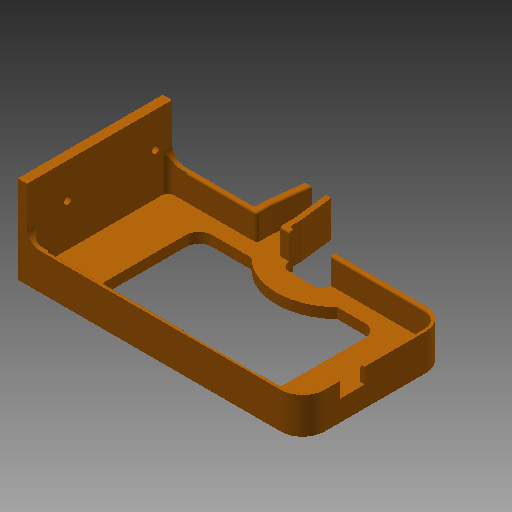
# Autodesk Inventor part: Phone_Cas
Saved by Autodesk Inventor 2019 (Build 230136000, 136)
## iProperties
Created: 2015-11-17
Part Number: Phone_Cas
Material: Generic
Document SubType Name: Modeling
Designer: Team Titanium
Density: 1 g/cm^3
Appearance: Orange
Author: Team Titanium
Autodesk Inventor part; units mm, degrees
ref_plane "YZ Plane" through (0, 0, 0) normal (1, 0, 0) x (0, 1, 0)
ref_plane "XZ Plane" through (0, 0, 0) normal (0, 1, 0) x (-1, 0, 0)
ref_plane "XY Plane" through (0, 0, 0) normal (0, 0, 1) x (1, 0, 0)
sketch "Sketch1" plane through (0, 0, 0) normal (0, 1, 0) x (-1, 0, 0)
  line L0 (67.1674, 24.5628) -> (-66.5636, 24.5628)
  line L1 (-66.5636, 24.5628) -> (-66.5636, -42.8742)
  line L2 (-66.5636, -42.8742) -> (67.1674, -42.8742)
  line L3 (67.1674, -42.8742) -> (67.1674, 24.5628)
  line L4 (69.1994, 26.5948) -> (-68.5956, 26.5948)
  line L5 (-68.5956, 26.5948) -> (-68.5956, -44.9062)
  line L6 (-68.5956, -44.9062) -> (69.1994, -44.9062)
  line L7 (69.1994, -44.9062) -> (69.1994, 26.5948)
  point P0 (0, 0)
  dimension "d0" = 133.731
  dimension "d1" = 67.437
  dimension "d2" = 2.032
  constraints: 16 end point, 4 parallel, 2 perpendicular, 1 horizontal, 3 other
  measures "d0" distance of L1.end L2.end
  measures "d1" distance of L2.end L0.start
  measures "d2" distance between parallel lines of L4 L0
extrude "Extrusion1" add sketch "Sketch1" along normal blind 12.7
sketch "Sketch2" plane through (0, 0, 0) normal (0, -1, 0) x (1, 0, 0)
  line L0 (68.5956, 26.5948) -> (68.5956, -44.9062) projected
  line L1 (68.5956, -44.9062) -> (-69.1994, -44.9062) projected
  line L2 (-69.1994, -44.9062) -> (-69.1994, 26.5948) projected
  line L3 (-69.1994, 26.5948) -> (68.5956, 26.5948) projected
  point P0 (0, 0)
extrude "Extrusion2" add sketch "Sketch2" along normal blind 5.08
fillet "Fillet1" radius 7.62 4 edges at (-67.1674, 6.35, -42.8742) (66.5636, 6.35, -42.8742) (-67.1674, 6.35, 24.5628) (66.5636, 6.35, 24.5628)
fillet "Fillet2" radius 10.795 4 edges at (-69.1994, 3.81, -44.9062) (68.5956, 3.81, -44.9062) (68.5956, 3.81, 26.5948) (-69.1994, 3.81, 26.5948)
sketch "Sketch3" plane through (0, 12.7, 0) normal (0, 1, 0) x (1, 0, 0)
  line L0 (57.8006, 44.9062) -> (-58.4044, 44.9062) projected
  line L1 (-59.5474, 42.8742) -> (58.9436, 42.8742) projected
  line L2 (-23.4286, 44.9062) -> (-12.7606, 44.9062)
  line L3 (-12.7606, 44.9062) -> (-12.7606, 42.8742)
  line L4 (-12.7606, 42.8742) -> (-23.4286, 42.8742)
  line L5 (-23.4286, 42.8742) -> (-23.4286, 44.9062)
  line L6 (-67.1674, -16.9428) -> (-67.1674, 35.2542) projected
  point P0 (0, 0)
  point P1 (-18.0946, 42.8742)
  dimension "d9" = 10.668
  dimension "d50" = 49.0728
  constraints: 8 end point, 2 parallel, 2 point on line, 1 horizontal, 1 midpoint, 1 perpendicular
  measures "d9" distance of L2.start L2.end
  measures "d50" distance from line of point (-18.095, 42.874) L6
extrude "Extrusion3" cut sketch "Sketch3" against normal up to surface (12.7 mm away)
sketch "Sketch4" plane through (0, 12.7, 0) normal (0, 1, 0) x (1, 0, 0)
  line L0 (-12.7606, 44.9062) -> (-12.7606, 50.6847)
  line L1 (-12.7606, 50.6847) -> (-14.8579, 67.7662)
  line L2 (-23.4286, 44.9062) -> (-23.4286, 50.6847)
  line L3 (-23.4286, 50.6847) -> (-21.3312, 67.7662)
  line L4 (-23.4286, 44.9062) -> (-58.4044, 44.9062) projected
  line L5 (-14.8579, 67.7662) -> (-11.6591, 67.7662)
  line L6 (-11.6591, 67.7662) -> (-9.5856, 50.8788)
  line L7 (57.8006, 44.9062) -> (-12.7606, 44.9062) projected
  line L8 (-9.5856, 44.9062) -> (-9.5856, 50.8788)
  line L9 (-21.3312, 67.7662) -> (-24.5301, 67.7662)
  line L10 (-24.5301, 67.7662) -> (-26.6036, 50.8788)
  line L11 (-26.6036, 50.8788) -> (-26.6036, 44.9062)
  line L12 (-67.1674, -16.9428) -> (-67.1674, 35.2542) projected
  point P0 (0, 0)
  dimension "d14" = 5.7785
  dimension "d15" = 22.86
  dimension "d17" = 3.175
  dimension "d18" = 3.175
  dimension "d19" = 3.175
  dimension "d20" = 3.175
  dimension "d45" = 173
  dimension "d46" = 173
  dimension "d47" = 6.4733
  constraints: 20 end point, 2 horizontal, 2 horizontal alignment, 2 perpendicular, 2 point on line, 2 vertical, 1 equal length, 1 parallel
  measures "d14" distance of L2.start L2.end
  measures "d15" distance from line of L3.end L4
  measures "d17" distance between parallel lines of L6 L1
  measures "d18" distance between parallel lines of L8 L0
  measures "d19" distance between parallel lines of L3 L10
  measures "d20" distance between parallel lines of L2 L11
  measures "d45" angle of L2 L3
  measures "d46" angle of L0 L1
  measures "d47" distance of L1.end L3.end
extrude "Extrusion4" add sketch "Sketch4" against normal up to surface (12.7 mm away)
sketch "Sketch5" plane through (0, -5.08, 0) normal (0, -1, 0) x (1, 0, 0)
  line L0 (-58.4044, -44.9062) -> (57.8006, -44.9062) projected
  line L1 (-26.6036, -50.8788) -> (-26.6036, -44.9062) projected
  line L2 (-24.5301, -67.7662) -> (-26.6036, -50.8788) projected
  line L3 (-9.5856, -50.8788) -> (-11.6591, -67.7662) projected
  line L4 (-9.5856, -44.9062) -> (-9.5856, -50.8788) projected
  line L5 (-24.5301, -67.7662) -> (-11.6591, -67.7662)
  point P0 (0, 0)
  constraints: 2 end point, 1 horizontal
extrude "Extrusion5" add sketch "Sketch5" against normal up to surface (5.08 mm away)
fillet "Fillet3" radius 1.524 2 edges at (-12.7606, 6.35, -42.8742) (-23.4286, 6.35, -42.8742)
fillet "Fillet4" radius 1.524 2 edges at (-26.6036, 3.81, -44.9062) (-9.5856, 3.81, -44.9062)
fillet "Fillet5" radius 1.016 15 edges at (-64.9355, 12.7, 22.331) (-67.1674, 12.7, -9.1557) (-64.9355, 12.7, -40.6423) (-42.25, 12.7, -42.8742) (-23.875, 12.7, -43.3205) (-23.4286, 12.7, -47.5414) (64.3318, 12.7, 22.331) (66.5636, 12.7, -9.1557) (64.3318, 12.7, -40.6423) (23.8535, 12.7, -42.8742) (-12.3142, 12.7, -43.3205) (-12.7606, 12.7, -47.5414) (-0.3019, 12.7, 24.5628) (-13.8093, 12.7, -59.2254) (-22.3799, 12.7, -59.2254)
sketch "Sketch6" plane through (0, 12.7, 0) normal (0, 1, 0) x (1, 0, 0)
  line L0 (-8.0616, 44.9062) -> (57.8006, 44.9062) projected
  line L1 (12.8426, 44.9062) -> (-7.4774, 44.9062)
  line L2 (-7.4774, 44.9062) -> (-7.4774, 38.5562)
  line L3 (-7.4774, 38.5562) -> (12.8426, 38.5562)
  line L4 (12.8426, 38.5562) -> (12.8426, 44.9062)
  line L5 (57.8006, -26.5948) -> (-58.4044, -26.5948) projected
  line L6 (-67.1674, -16.9428) -> (-67.1674, 35.2542) projected
  point P0 (0, 0)
  point P1 (2.6826, 38.5562)
  dimension "d29" = 6.35
  dimension "d30" = 69.85
  dimension "d61" = 20.32
  constraints: 8 end point, 2 parallel, 1 horizontal, 1 midpoint, 1 perpendicular, 1 point on line
  measures "d29" distance between parallel lines of L3 L0
  measures "d30" distance from line of point (2.683, 38.556) L6
  measures "d61" distance of L2.end L3.end
extrude "Extrusion6" cut sketch "Sketch6" against normal through all
fillet "Fillet6" radius 4.064 2 edges at (-7.4774, -2.54, -38.5562) (12.8426, -2.54, -38.5562)
sketch "Sketch8" plane through (0, 0, 0) normal (0, 1, 0) x (1, 0, 0)
  line L0 (-44.3074, -16.9428) -> (43.7036, -16.9428)
  line L1 (43.7036, -16.9428) -> (43.7036, 35.2542)
  line L2 (43.7036, 35.2542) -> (-44.3074, 35.2542)
  line L3 (-44.3074, 35.2542) -> (-44.3074, -16.9428)
  line L4 (-67.1674, -16.9428) -> (-67.1674, 35.2542) projected
  line L5 (66.5636, 35.2542) -> (66.5636, -16.9428) projected
  line L6 (58.9436, -24.5628) -> (-59.5474, -24.5628) projected
  line L7 (-11.2366, 42.8742) -> (58.9436, 42.8742) projected
  point P0 (0, 0)
  point P1 (12.8426, -24.5628)
  point P2 (12.8426, 42.8742)
  dimension "d53" = 22.86
  dimension "d54" = 22.86
  dimension "d55" = 7.62
  dimension "d56" = 7.62
  constraints: 8 end point, 2 parallel, 1 horizontal, 1 perpendicular
  measures "d53" distance between parallel lines of L3 L4
  measures "d54" distance between parallel lines of L1 L5
  measures "d55" distance between parallel lines of L0 L6
  measures "d56" distance between parallel lines of L2 L7
extrude "Extrusion8" cut sketch "Sketch8" against normal through all
fillet "Fillet7" radius 6.35 4 edges at (-44.3074, -2.54, -35.2542) (-44.3074, -2.54, 16.9428) (43.7036, -2.54, 16.9428) (43.7036, -2.54, -35.2542)
sketch "Sketch10" plane through (0, 0, 0) normal (0, 1, 0) x (1, 0, 0)
  line L0 (-37.9574, -16.9428) -> (37.3536, -16.9428) projected
  line L1 (37.3536, 35.2542) -> (-37.9574, 35.2542) projected
  arc A0 (-18.5377, 35.2542) -> (23.6849, 35.2542) centre (2.5736, 56.3248) ccw
  point P0 (0, 0)
  constraints: 2 point on circle, 2 point on line, 1 centre point
extrude "Extrusion10" add sketch "Sketch10" against normal up to surface (5.08 mm away)
sketch "Sketch11" plane through (0, 12.7, 0) normal (0, 1, 0) x (1, 0, 0)
  line L0 (64.9731, -8.3068) -> (68.5956, -8.3068)
  line L1 (68.5956, -8.3068) -> (68.5956, 3.8852)
  line L2 (68.5956, 3.8852) -> (64.9731, 3.8852)
  line L3 (64.9731, 3.8852) -> (64.9731, -8.3068)
  line L4 (58.9436, -24.5628) -> (-59.5474, -24.5628) projected
  line L5 (68.5956, -15.7998) -> (68.5956, 34.1112) projected
  point P0 (0, 0)
  point P1 (64.9731, -2.2108)
  dimension "d62" = 12.192
  dimension "d63" = 22.352
  dimension "d72" = 0
  constraints: 8 end point, 2 parallel, 1 horizontal, 1 midpoint, 1 perpendicular
  measures "d62" distance of L2.end L0.start
  measures "d63" distance from line of L4 point (64.973, -2.211)
  measures "d72" distance between parallel lines of L5 L1
extrude "Extrusion11" cut sketch "Sketch11" against normal blind 7.62
sketch "Sketch13" plane through (0, 12.7, 0) normal (0, 1, 0) x (1, 0, 0)
  line L0 (20.9706, -25.5788) -> (46.3706, -25.5788)
  line L1 (46.3706, -25.5788) -> (46.3706, -24.5628)
  line L2 (46.3706, -24.5628) -> (20.9706, -24.5628)
  line L3 (20.9706, -24.5628) -> (20.9706, -25.5788)
  line L4 (-59.5474, -24.5628) -> (58.9436, -24.5628) projected
  line L5 (68.5956, -15.7998) -> (68.5956, -8.3068) projected
  line L6 (-58.4044, -26.5948) -> (57.8006, -26.5948) projected
  point P0 (0, 0)
  dimension "d73" = 0
  dimension "d74" = 22.225
  dimension "d75" = 25.4
  dimension "d77" = 1.016
  constraints: 8 end point, 2 parallel, 1 horizontal, 1 perpendicular
  measures "d73" distance between parallel lines of L4 L2
  measures "d74" distance between parallel lines of L5 L1
  measures "d75" distance between parallel lines of L3 L1
  measures "d77" distance between parallel lines of L6 L0
extrude "Extrusion13" cut sketch "Sketch13" against normal up to surface (12.7 mm away)
thicken "Thicken1" operation add thickness 12.7 both sides no extend neighbours yes toward (-1, 0, 0) faces at (20.9706, 8.128, 25.2402)
sketch "Sketch14" plane through (-69.1994, -5.08, 15.7998) normal (-1, 0, 0) x (0, 0, 1)
  line L0 (0, 17.78) -> (0, 0) projected
  line L1 (-49.911, 17.78) -> (0, 17.78) projected
  line L2 (-49.911, 0) -> (-49.911, 17.78) projected
  line L3 (0, 0) -> (-49.911, 0) projected
  point P0 (-15.7998, 5.08)
extrude "Extrusion14" add sketch "Sketch14" along normal blind 2.54
sketch "Sketch15" plane through (0, 12.7, 0) normal (0, 1, 0) x (1, 0, 0)
  line L0 (68.5956, -8.3068) -> (67.5796, -8.3068) projected
  line L1 (67.5796, -16.9428) -> (67.5796, -8.3068) projected
  arc A0 (58.9436, -25.5788) -> (67.5796, -16.9428) centre (58.9436, -16.9428) ccw projected
  line L2 (46.3706, -25.5788) -> (58.9436, -25.5788) projected
  line L3 (8.2706, -25.5788) -> (46.3706, -25.5788) projected
  line L4 (-59.5474, -25.5788) -> (8.2706, -25.5788) projected
  arc A1 (-68.1834, -16.9428) -> (-59.5474, -25.5788) centre (-59.5474, -16.9428) ccw projected
  line L5 (-68.1834, 35.2542) -> (-68.1834, -16.9428) projected
  arc A2 (-59.5474, 43.8902) -> (-68.1834, 35.2542) centre (-59.5474, 35.2542) ccw projected
  line L6 (-24.9526, 43.8902) -> (-59.5474, 43.8902) projected
  arc A3 (-24.9526, 43.8902) -> (-24.4446, 44.3982) centre (-24.9526, 44.3982) ccw projected
  line L7 (-24.4446, 50.7468) -> (-24.4446, 44.3982) projected
  line L8 (-22.3549, 67.7662) -> (-24.4446, 50.7468) projected
  line L9 (-22.3549, 67.7662) -> (-24.5301, 67.7662) projected
  line L10 (-24.5301, 67.7662) -> (-26.6036, 50.8788) projected
  line L11 (-26.6036, 50.8788) -> (-26.6036, 46.4302) projected
  arc A4 (-28.1276, 44.9062) -> (-26.6036, 46.4302) centre (-28.1276, 46.4302) ccw projected
  line L12 (-28.1276, 44.9062) -> (-58.4044, 44.9062) projected
  arc A5 (-58.4044, 44.9062) -> (-69.1994, 34.1112) centre (-58.4044, 34.1112) ccw projected
  line L13 (-69.1994, 34.1112) -> (-71.7394, 34.1112) projected
  line L14 (-71.7394, -15.7998) -> (-71.7394, 34.1112) projected
  line L15 (-69.1994, -15.7998) -> (-71.7394, -15.7998) projected
  arc A6 (-69.1994, -15.7998) -> (-58.4044, -26.5948) centre (-58.4044, -15.7998) ccw projected
  line L16 (-58.4044, -26.5948) -> (57.8006, -26.5948) projected
  arc A7 (57.8006, -26.5948) -> (68.5956, -15.7998) centre (57.8006, -15.7998) ccw projected
  line L17 (68.5956, -15.7998) -> (68.5956, -8.3068) projected
  line L18 (-71.7394, 34.1112) -> (-71.7394, -15.7998) projected
  line L19 (-68.1834, 35.2542) -> (-68.1834, -16.9428) projected
  line L20 (-71.7394, 34.1112) -> (-68.1834, 34.1112)
  line L21 (-68.1834, -15.7998) -> (-71.7394, -15.7998)
  line L22 (-71.7394, -15.7998) -> (-71.7394, 34.1112)
  line L23 (-67.1674, 35.2542) -> (-68.1834, 35.2542) projected
  line L24 (-68.1834, 35.2542) -> (-68.1834, -16.9428) projected
  line L25 (-67.1674, -16.9428) -> (-68.1834, -16.9428) projected
  line L26 (-67.1674, -16.9428) -> (-67.1674, 35.2542) projected
  line L27 (-69.1994, -15.7998) -> (-71.7394, -15.7998) projected
  line L28 (-67.1674, 35.2542) -> (-67.1674, -16.9428) projected
  line L29 (-71.7394, -15.7998) -> (-67.1674, -15.7998)
  line L30 (-67.1674, -15.7998) -> (-67.1674, 34.1112)
  line L31 (-67.1674, 34.1112) -> (-71.7394, 34.1112)
  line L32 (-71.7394, 34.1112) -> (-71.7394, -15.7998)
  line L33 (-68.1834, 34.1112) -> (-68.1834, 29.5392)
  line L34 (-71.7394, -15.7998) -> (-68.1834, -15.7998)
  line L35 (-67.1674, 34.1112) -> (-68.1834, 34.1112)
  point P0 (0, 0)
  dimension "d88" = 4.572
  dimension "d89" = 3.556
  constraints: 20 end point, 4 parallel, 2 collinear, 2 horizontal, 2 perpendicular, 2 point on line, 1 point on circle
  measures "d88" distance between parallel lines of L26 L14
  measures "d89" distance of L13.end L20.end
fillet "Fillet10" radius 2.54 2 edges at (-71.7394, 3.81, 15.7998) (-71.7394, 3.81, -34.1112)
extrude "Extrusion17" add sketch "Sketch15" along normal blind 15.875 and the other way blind 31.75 contours L15 L14 L13 L20 L5 L21 | L5 L31 L26 L29
fillet "Fillet11" radius 3.175 1 edges at (-67.1674, -5.08, -9.1557)
thicken "Thicken2" operation add thickness 9.525 both sides no extend neighbours yes toward (0, 1, 0) faces at (-70.2154, 28.575, -0.8372)
thicken "Thicken3" operation add thickness 13.97 both sides no extend neighbours yes toward (0, 1, 0) faces at (-70.2154, -19.05, -0.8372)
thicken "Thicken4" operation add thickness 3.175 both sides no extend neighbours yes toward (1, 0, 0) faces at (-67.1674, -7.1967, -0.8372)
sketch "Sketch17" plane through (-68.1834, 12.7, -34.1112) normal (0, 0, -1) x (-1, 0, 0)
  line L0 (-1.016, -1.016) -> (-1.016, 25.4) projected
  line L1 (3.556, -17.78) -> (3.556, 25.4) projected
  line L2 (-1.016, 25.4) -> (3.556, 25.4)
  line L3 (3.556, 25.4) -> (3.556, -17.78)
  line L4 (3.556, -17.78) -> (-1.016, -17.78)
  line L5 (-1.016, -17.78) -> (-1.016, 25.4)
  point P0 (-68.1834, -12.7)
  constraints: 8 end point, 2 parallel, 1 horizontal, 1 perpendicular
extrude "Extrusion18" add sketch "Sketch17" along normal up to surface (10.795 mm away)
sketch "Sketch18" plane through (-28.1276, 12.7, -44.9062) normal (0, 0, -1) x (-1, 0, 0)
  line L0 (0, 0) -> (30.2768, 0) projected
  line L1 (30.2768, 0) -> (39.0398, 0)
  line L2 (39.0398, 0) -> (39.0398, -17.78)
  line L3 (39.0398, -17.78) -> (30.2768, -17.78)
  line L4 (30.2768, -17.78) -> (30.2768, 0)
  point P0 (-28.1276, -12.7)
  constraints: 8 end point, 2 parallel, 1 horizontal, 1 perpendicular
extrude "Extrusion19" add sketch "Sketch18" against normal up to surface (4.4909 mm away)
sketch "Sketch19" plane through (0, 12.7, 0) normal (0, 1, 0) x (1, 0, 0)
  line L0 (-58.4044, 42.8742) -> (-24.9526, 42.8742) projected
  arc A0 (-65.1534, 40.4153) -> (-67.1674, 35.2542) centre (-59.5474, 35.2542) ccw projected
  line L1 (-58.4044, 42.8742) -> (-65.1534, 42.8742)
  line L2 (-65.1534, 42.8742) -> (-65.1534, 40.4153)
  line L3 (-65.1534, 40.4153) -> (-58.4044, 40.4153)
  line L4 (-58.4044, 40.4153) -> (-58.4044, 42.8742)
  line L5 (-58.4044, 42.8742) -> (-67.1674, 42.8742)
  line L6 (-67.1674, 42.8742) -> (-67.1674, 35.2542)
  line L7 (-67.1674, 35.2542) -> (-58.4044, 35.2542)
  line L8 (-58.4044, 35.2542) -> (-58.4044, 42.8742)
  point P0 (0, 0)
  constraints: 16 end point, 4 parallel, 2 horizontal, 2 perpendicular
extrude "Extrusion20" cut sketch "Sketch19" against normal up to surface (12.7 mm away)
sketch "Sketch20" plane through (-69.1994, 12.7, 15.7998) normal (0, 0, 1) x (1, 0, 0)
  line L0 (-2.54, 25.4) -> (-2.54, -17.78) projected
  line L1 (10.795, -17.78) -> (0, -17.78) projected
  line L2 (-2.54, 25.4) -> (2.035, 25.4)
  line L3 (2.035, 25.4) -> (2.035, -17.78)
  line L4 (2.035, -17.78) -> (-2.54, -17.78)
  line L5 (-2.54, -17.78) -> (-2.54, 25.4)
  point P0 (69.1994, -12.7)
  constraints: 8 end point, 2 parallel, 1 horizontal, 1 perpendicular, 1 point on line
extrude "Extrusion21" add sketch "Sketch20" along normal up to surface (10.795 mm away)
sketch "Sketch21" plane through (-58.4044, 12.7, 26.5948) normal (0, 0, 1) x (1, 0, 0)
  line L0 (0, -17.78) -> (-8.76, -17.78) projected
  line L1 (-8.763, 0) -> (0, 0) projected
  line L2 (0, -17.78) -> (-8.763, -17.78)
  line L3 (-8.763, -17.78) -> (-8.763, 0)
  line L4 (-8.763, 0) -> (0, 0)
  line L5 (0, 0) -> (0, -17.78)
  point P0 (58.4044, -12.7)
  constraints: 8 end point, 2 parallel, 1 horizontal, 1 perpendicular
extrude "Extrusion22" add sketch "Sketch21" against normal up to surface (9.4387 mm away)
sketch "Sketch22" plane through (0, 12.7, 0) normal (0, 1, 0) x (1, 0, 0)
  line L0 (-58.4044, -25.5788) -> (-58.4044, -17.1562) projected
  line L1 (-58.4044, -24.5538) -> (-67.1644, -24.5538)
  line L2 (-67.1644, -24.5538) -> (-67.1644, -17.1562)
  line L3 (-67.1644, -17.1562) -> (-58.4044, -17.1562)
  line L4 (-58.4044, -17.1562) -> (-58.4044, -24.5538)
  point P0 (0, 0)
  constraints: 8 end point, 2 parallel, 1 horizontal, 1 perpendicular, 1 point on line
extrude "Extrusion23" cut sketch "Sketch22" against normal up to surface (12.7 mm away)
fillet "Fillet12" radius 6.35 2 edges at (-67.1674, 12.7, -43.8902) (-67.1644, 12.7, 25.5743)
fillet "Fillet13" radius 3.175 4 edges at (-67.1644, 15.875, 24.5538) (-67.1644, 6.35, 24.5538) (-67.1674, 15.875, -42.8742) (-67.1674, 6.35, -42.8742)
sketch "Sketch23" plane through (-71.7394, -5.08, 15.7998) normal (-1, 0, 0) x (0, 0, 1)
  line L0 (10.795, 43.18) -> (-60.706, 43.18) projected
  line L1 (-60.706, 43.18) -> (-60.706, 0) projected
  line L2 (-60.706, 0) -> (10.795, 0) projected
  line L3 (10.795, 0) -> (10.795, 43.18) projected
  point P0 (-15.7998, 5.08)
  point P1 (-52.578, 25.9588)
  point P2 (-9.2456, 25.9588)
  dimension "d118" = 17.2212
  dimension "d119" = 17.2212
  dimension "d120" = 8.128
  dimension "d121" = 51.4604
  measures "d118" distance from line of L0 point (-52.578, 25.959)
  measures "d119" distance from line of L0 point (-9.246, 25.959)
  measures "d120" distance from line of L1 point (-52.578, 25.959)
  measures "d121" distance from line of point (-9.246, 25.959) L1
hole "Hole1" at (-71.7394, 20.8788, -36.7782) at (-71.7394, 20.8788, 6.5542) direction (1, 0, 0) diameter 3.556 depth 25.4 tip angle 118
sketch "Sketch12" plane through (0, 0, 0) normal (0, 1, 0) x (1, 0, 0)
  line L0 (-37.1264, 29.2031) -> (-37.1264, 48.6718)
  line L1 (-37.1264, 48.6718) -> (-76.0638, 48.6718)
  line L2 (-76.0638, 48.6718) -> (-76.0638, -33.2779)
  line L3 (-76.0638, -33.2779) -> (73.5736, -33.2779)
  line L4 (73.5736, -33.2779) -> (73.5736, -28.0712)
  line L5 (73.5736, -28.0712) -> (56.8215, -28.0712)
  line L6 (56.8215, -28.0712) -> (56.8215, 13.3564)
  line L7 (56.8215, 13.3564) -> (73.5736, 13.3564)
  line L8 (73.5736, 13.3564) -> (73.5736, 51.8411)
  line L9 (73.5736, 51.8411) -> (0, 53.4258)
  line L10 (0, 53.4258) -> (0, 21.4966)
  line L11 (0, 21.4966) -> (-37.1264, 29.2031)
  point P0 (0, 0)
  constraints: 24 end point, 7 perpendicular, 2 point on line, 1 parallel, 1 vertical
equation "\"d119\" = d118"
body "Solid1"
